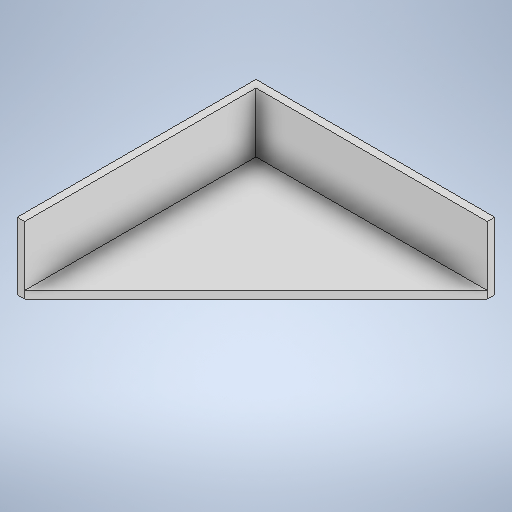
# Autodesk Inventor part: Right Angle Gig
Saved by Autodesk Inventor 2025.1 (Build 291241020, 241B)
## iProperties
Created: 2025-01-27
Part Number: Right Angle Gig
Material: Generic
Document SubType Name: Modeling
Designer: dpseu
Density: 1 g/cm^3
Appearance: Default
Author: dpseu
Autodesk Inventor part; units mm, degrees
ref_plane "YZ Plane" through (0, 0, 0) normal (1, 0, 0) x (0, 1, 0)
ref_plane "XZ Plane" through (0, 0, 0) normal (0, 1, 0) x (-1, 0, 0)
ref_plane "XY Plane" through (0, 0, 0) normal (0, 0, 1) x (1, 0, 0)
sketch "Sketch1" plane through (0, 0, 0) normal (0, 1, 0) x (-1, 0, 0)
  line L0 (0, 0) -> (101.6, 0)
  line L1 (101.6, 0) -> (101.6, -3.175)
  line L2 (101.6, -3.175) -> (3.175, -3.175)
  line L3 (0, -3.175) -> (0, 0)
  line L4 (0, 0) -> (3.175, 0)
  line L5 (3.175, -3.175) -> (3.175, -101.6)
  line L6 (3.175, -101.6) -> (0, -101.6)
  line L7 (0, -101.6) -> (0, 0)
  dimension "d0" = 101.6
  dimension "d1" = 3.175
  dimension "d2" = 3.175
  dimension "d3" = 101.6
  constraints: 16 end point, 4 parallel, 2 horizontal, 2 perpendicular
  measures "d0" distance of L1.end L3.start
  measures "d1" distance of L0.end L1.end
  measures "d2" distance of L5.end L6.end
  measures "d3" distance of L4.end L5.end
extrude "Extrusion1" add sketch "Sketch1" along normal blind 28.575
sketch "Sketch2" plane through (0, 0, 0) normal (0, -1, 0) x (1, 0, 0)
  line L0 (-3.175, -101.6) -> (-3.175, -3.175) projected
  line L1 (-3.175, -3.175) -> (-101.6, -3.175) projected
  line L2 (-3.175, -101.6) -> (-101.6, -3.175)
  point P0 (0, 0)
  constraints: 2 end point
extrude "Extrusion2" add sketch "Sketch2" against normal blind 3.175
body "Solid1"
